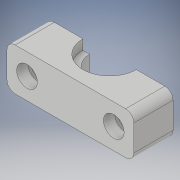
# Autodesk Inventor part: e3D_V6_Bowden_Clamp_01
Saved by Autodesk Inventor 2019.4 (Build 234330000, 330)
## iProperties
Created: 2019-11-21
Part Number: e3D_V6_Bowden_Clamp_01
Material: Generic
Document SubType Name: Modeling
Designer: frogm
Density: 1 g/cm^3
Appearance: Default
Author: frogm
Autodesk Inventor part; units mm, degrees
ref_plane "YZ Plane" through (0, 0, 0) normal (1, 0, 0) x (0, 1, 0)
ref_plane "XZ Plane" through (0, 0, 0) normal (0, 1, 0) x (-1, 0, 0)
ref_plane "XY Plane" through (0, 0, 0) normal (0, 0, 1) x (1, 0, 0)
sketch "Base Sketch" plane through (0, 0, 0) normal (0, 0, 1) x (1, 0, 0)
  line L0 (-16.55, 6.35) -> (16.55, 6.35)
  line L1 (19, 3.9) -> (19, -3.9)
  line L2 (16.55, -6.35) -> (-16.55, -6.35)
  line L3 (-19, -3.9) -> (-19, 3.9)
  line L4 (0, 9.6004) -> (0, -9.6004) construction
  line L5 (-27.3104, 0) -> (27.3104, 0) construction
  arc A0 (19, 3.9) -> (16.55, 6.35) centre (16.55, 3.9) ccw
  arc A1 (-16.55, 6.35) -> (-19, 3.9) centre (-16.55, 3.9) ccw
  arc A2 (-19, -3.9) -> (-16.55, -6.35) centre (-16.55, -3.9) ccw
  arc A3 (16.55, -6.35) -> (19, -3.9) centre (16.55, -3.9) ccw
  point P0 (0, 0)
  point P1 (19, -6.35)
  point P2 (-19, -6.35)
  point P3 (0, 6.35)
  point P4 (19, 0)
  dimension "d0" = 38
  dimension "d2" = 2.45
  dimension "d3" = 12.7
  constraints: 8 end point, 8 point on circle, 8 tangent, 6 point on line, 4 centre point, 3 equal radius, 2 midpoint, 2 parallel, 1 horizontal, 1 perpendicular
  measures "d0" distance of point (19, -6.35) point (-19, -6.35)
  measures "d2" radius of A0
  measures "d3" distance between parallel lines of L2 L0
extrude "Base Extrusion (11.75)" add sketch "Base Sketch" against normal blind 11.75
sketch "Screw Holes Sketch" plane through (0, 0, 0) normal (0, 0, 1) x (1, 0, 0)
  line L0 (0, 8.89) -> (0, -8.89) construction
  line L1 (-26.6, 0) -> (26.6, 0) construction
  circle A0 centre (-13, 0) radius 2.05
  circle A1 centre (-13, 0) radius 3.1
  circle A2 centre (13, 0) radius 2.05
  circle A3 centre (13, 0) radius 3.1
  point P0 (0, 0)
  dimension "d6" = 4.1
  dimension "d7" = 13
  dimension "d8" = 6.2
  constraints: 4 centre point, 2 coincident, 2 symmetric about line, 1 point on line, 2 other
  measures "d6" diameter of A0
  measures "d7" distance from line of L0 A0.centre
  measures "d8" diameter of A1
extrude "Screw Holes Extrusion (To)" cut sketch "Screw Holes Sketch" against normal up to surface (11.75 mm away) contours A0 | A2
extrude "Screw Counterbores Extrusion (3.4)" cut sketch "Screw Holes Sketch" against normal blind 3.4
sketch "Heatsink Arcs Sketch" plane through (-16.55, 6.35, 0) normal (0, 1, 0) x (1, 0, 0)
  arc A0 (10.55, 11.75) -> (22.55, 11.75) centre (16.55, 11.75) ccw
  arc A1 (8.55, 11.75) -> (24.55, 11.75) centre (16.55, 11.75) ccw
  line L0 (8.55, 11.75) -> (10.55, 11.75)
  line L1 (22.55, 11.75) -> (24.55, 11.75)
  line L2 (10.55, 11.75) -> (22.55, 11.75)
  point P0 (16.55, 0)
  dimension "d13" = 6
  dimension "d14" = 8
  constraints: 6 end point, 4 point on circle, 2 centre point, 2 coincident
  measures "d13" radius of A0
  measures "d14" radius of A1
extrude "Top Outer Arc Extrusion (3)" cut sketch "Heatsink Arcs Sketch" against normal blind 3 contours A0 L1 A1 L0
extrude "Inner Arc Extrusion (Through)" cut sketch "Heatsink Arcs Sketch" against normal up to surface (12.7 mm away) contours L2 A0
ref_plane "Lower Outer Arc Plane (9)" through (-16.55, -2.65, 0) normal (0, 1, 0) x (1, 0, 0)
sketch "Sketch4" plane through (-16.55, -2.65, 0) normal (0, 1, 0) x (1, 0, 0)
  arc A0 (8.55, 11.75) -> (24.55, 11.75) centre (16.55, 11.75) ccw projected
  arc A1 (10.55, 11.75) -> (22.55, 11.75) centre (16.55, 11.75) ccw projected
  line L0 (22.55, 11.75) -> (24.55, 11.75) projected
  line L1 (8.55, 11.75) -> (10.55, 11.75) projected
  point P0 (16.55, 0)
extrude "Bottom Outer Arc Extrusion (3.7)" cut sketch "Sketch4" against normal up to surface (3.7 mm away)
body "Solid1"
